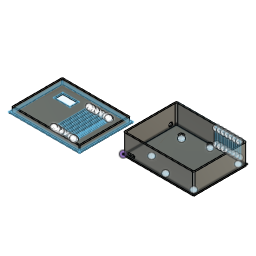
Enclosure temperature control box v10 (Autodesk Fusion 360 design; units mm, degrees)
Autodesk Fusion 360 part; units mm, degrees
sketch "Sketch1" plane through (0, 0, 0) normal (0, 0, 1) x (1, 0, 0)
  line L0 (0, 0) -> (110, 0)
  line L1 (110, 0) -> (110, 83)
  line L2 (110, 83) -> (0, 83)
  line L3 (0, 83) -> (0, 0)
  circle A0 centre (24.6, 66.3) radius 1.8
  circle A1 centre (24.6, 19.6) radius 1.8
  circle A2 centre (59.2, 6.8) radius 1.5
  circle A3 centre (103.2, 6.8) radius 1.5
  circle A4 centre (103.2, 76.2) radius 1.5
  circle A5 centre (59.2, 76.2) radius 1.5
  line L4 (2, 81) -> (108, 81)
  line L5 (108, 81) -> (108, 2)
  line L6 (108, 2) -> (2, 2)
  line L7 (2, 2) -> (2, 81)
  circle A6 centre (24.6, 66.3) radius 3.8
  circle A7 centre (24.6, 19.6) radius 3.8
  circle A8 centre (59.2, 76.2) radius 3.5
  circle A9 centre (103.2, 76.2) radius 3.5
  circle A10 centre (59.2, 6.8) radius 3.5
  circle A11 centre (103.2, 6.8) radius 3.5
  dimension "d1" = 110
  dimension "d2" = 83
  dimension "d10" = 3.6
  dimension "d13" = 3.6
  dimension "d16" = 3
  dimension "d19" = 3
  dimension "d22" = 3
  dimension "d25" = 3
  dimension "d28" = 106
  dimension "d29" = 79
  dimension "d30" = 2
  dimension "d31" = 2
  dimension "d40" = 7.6
  dimension "d41" = 7.6
  dimension "d42" = 7
  dimension "d43" = 7
  dimension "d44" = 7
  dimension "d45" = 7
  constraint horizontal L0
  constraint vertical L1
  constraint horizontal L2
  constraint vertical L3
  constraint coincident L0.start L3.end
  constraint horizontal L4
  constraint vertical L5
  constraint horizontal L6
  constraint vertical L7
  constraint concentric A0 A6
  constraint concentric A1 A7
  constraint concentric A5 A8
  constraint concentric A4 A9
  constraint concentric A2 A10
  constraint concentric A3 A11
  measures "d1" distance of L0.start L0.end
  measures "d2" distance of L0.start L2.end
  measures "d10" diameter of A0
  measures "d13" diameter of A1
  measures "d16" diameter of A2
  measures "d19" diameter of A3
  measures "d22" diameter of A4
  measures "d25" diameter of A5
  measures "d28" distance of L4.start L4.end
  measures "d29" distance of L4.start L6.end
  measures "d30" distance of L2 L4
  measures "d31" distance of L1 L5
  measures "d40" diameter of A6
  measures "d41" diameter of A7
  measures "d42" diameter of A8
  measures "d43" diameter of A9
  measures "d44" diameter of A10
  measures "d45" diameter of A11
extrude "Extrude4" add sketch "Sketch1" against normal blind 3 contours L0 L1 L2 L3 | A0 | A1 | A2 | A3 | A4 | A5 | L4 L5 L6 L7 | A6 | A7 | A8 | A9 | A10 | A11 makes body 1
extrude "Extrude5" add sketch "Sketch1" along normal blind 5 contours A6 | A7 | A8 | A9 | A10 | A11 bodies 1
extrude "Extrude6" add sketch "Sketch1" along normal blind 30 contours L0 L1 L2 L3 bodies 1
fillet "Fillet2" radius 2 4 edges at (110, 0, 13.5) (110, 83, 13.5) (0, 83, 13.5) (0, 0, 13.5) on bodies 1
fillet "Fillet3" radius 2 4 edges at (2, 2, 15) (108, 2, 15) (108, 81, 15) (2, 81, 15) on bodies 1
fillet "Fillet4" radius 1 8 edges at (109.4142, 82.4142, -3) (110, 41.5, -3) (109.4142, 0.5858, -3) (55, 0, -3) (0.5858, 0.5858, -3) (0, 41.5, -3) (0.5858, 82.4142, -3) (55, 83, -3) on bodies 1
sketch "Sketch2" plane through (0, 83, 0) normal (0, 1, 0) x (-1, 0, 0)
  line L0 (-108, -2) -> (-2, -2)
  line L1 (-2, -2) -> (-2, 30)
  line L2 (-2, 30) -> (-108, 30)
  line L3 (-108, 30) -> (-108, -2)
  line L4 (-97.0499, 25) -> (-97.0499, 3)
  line L5 (-100.0499, 3) -> (-100.0499, 25)
  arc A0 (-97.0499, 25) -> (-100.0499, 25) centre (-98.5499, 25) ccw
  arc A1 (-100.0499, 3) -> (-97.0499, 3) centre (-98.5499, 3) ccw
  line L6 (-94.0499, 3) -> (-94.0499, 25)
  line L7 (-91.0499, 25) -> (-91.0499, 3)
  arc A2 (-91.0499, 25) -> (-94.0499, 25) centre (-92.5499, 25) ccw
  arc A3 (-94.0499, 3) -> (-91.0499, 3) centre (-92.5499, 3) ccw
  line L8 (-88.0499, 3) -> (-88.0499, 25)
  line L9 (-85.0499, 25) -> (-85.0499, 3)
  arc A4 (-85.0499, 25) -> (-88.0499, 25) centre (-86.5499, 25) ccw
  arc A5 (-88.0499, 3) -> (-85.0499, 3) centre (-86.5499, 3) ccw
  line L10 (-82.0499, 3) -> (-82.0499, 25)
  line L11 (-79.0499, 25) -> (-79.0499, 3)
  arc A6 (-79.0499, 25) -> (-82.0499, 25) centre (-80.5499, 25) ccw
  arc A7 (-82.0499, 3) -> (-79.0499, 3) centre (-80.5499, 3) ccw
  line L12 (-76.0499, 3) -> (-76.0499, 25)
  line L13 (-73.0499, 25) -> (-73.0499, 3)
  arc A8 (-73.0499, 25) -> (-76.0499, 25) centre (-74.5499, 25) ccw
  arc A9 (-76.0499, 3) -> (-73.0499, 3) centre (-74.5499, 3) ccw
  line L14 (-70.0499, 3) -> (-70.0499, 25)
  line L15 (-67.0499, 25) -> (-67.0499, 3)
  arc A10 (-67.0499, 25) -> (-70.0499, 25) centre (-68.5499, 25) ccw
  arc A11 (-70.0499, 3) -> (-67.0499, 3) centre (-68.5499, 3) ccw
  line L16 (-64.0499, 3) -> (-64.0499, 25)
  line L17 (-61.0499, 25) -> (-61.0499, 3)
  arc A12 (-61.0499, 25) -> (-64.0499, 25) centre (-62.5499, 25) ccw
  arc A13 (-64.0499, 3) -> (-61.0499, 3) centre (-62.5499, 3) ccw
  dimension "d60" = 1.5
  dimension "d61" = 1.5
  dimension "d62" = 1.5
  dimension "d63" = 1.5
  dimension "d64" = 1.5
  dimension "d65" = 1.5
  dimension "d66" = 1.5
  dimension "d67" = 1.5
  dimension "d68" = 1.5
  dimension "d69" = 1.5
  dimension "d70" = 1.5
  dimension "d71" = 1.5
  dimension "d72" = 1.5
  dimension "d73" = 1.5
  dimension "d74" = 5
  dimension "d75" = 5
  dimension "d76" = 5
  dimension "d77" = 5
  dimension "d78" = 5
  dimension "d79" = 5
  dimension "d80" = 5
  dimension "d81" = 3
  dimension "d82" = 3
  dimension "d83" = 3
  dimension "d84" = 22
  dimension "d85" = 3
  dimension "d86" = 3
  dimension "d87" = 3
  constraint vertical L4
  constraint vertical L5
  constraint tangent L5 A0
  constraint tangent L4 A0
  constraint vertical L7
  constraint vertical L6
  constraint tangent L6 A2
  constraint tangent L7 A2
  constraint vertical L9
  constraint vertical L8
  constraint tangent L8 A4
  constraint tangent L9 A4
  constraint vertical L11
  constraint vertical L10
  constraint tangent L10 A6
  constraint tangent L11 A6
  constraint vertical L13
  constraint vertical L12
  constraint tangent L12 A8
  constraint tangent L13 A8
  constraint vertical L15
  constraint vertical L14
  constraint tangent L14 A10
  constraint tangent L15 A10
  constraint vertical L17
  constraint vertical L16
  constraint tangent L16 A12
  constraint tangent L17 A12
  measures "d60" radius of A0
  measures "d61" radius of A1
  measures "d62" radius of A2
  measures "d63" radius of A3
  measures "d64" radius of A4
  measures "d65" radius of A5
  measures "d66" radius of A6
  measures "d67" radius of A7
  measures "d68" radius of A8
  measures "d69" radius of A9
  measures "d70" radius of A10
  measures "d71" radius of A11
  measures "d72" radius of A12
  measures "d73" radius of A13
  measures "d74" distance of L2 A0.centre
  measures "d75" distance of L2 A2.centre
  measures "d76" distance of L2 A4.centre
  measures "d77" distance of L2 A6.centre
  measures "d78" distance of L2 A8.centre
  measures "d79" distance of L2 A10.centre
  measures "d80" distance of L2 A12.centre
  measures "d81" distance of L4 L6
  measures "d82" distance of L7 L8
  measures "d83" distance of L9 L10
  measures "d84" distance of L12.end L12.start
  measures "d85" distance of L11 L12
  measures "d86" distance of L13 L14
  measures "d87" distance of L15 L16
extrude "Extrude8" cut sketch "Sketch2" along normal mid plane 5.5 contours L4 L5 A0 A1 | L6 L7 A2 A3 | L8 L9 A4 A5 | L10 L11 A6 A7 | L12 L13 A8 A9 | L14 L15 A10 A11 | L16 L17 A12 A13 bodies 1
sketch "Sketch3" plane through (0, 0, 0) normal (0, 0, 1) x (1, 0, 0)
  line L0 (-146.1549, 50.841) -> (-36.1549, 50.841)
  line L1 (-36.1549, 50.841) -> (-36.1549, -32.159)
  line L2 (-36.1549, -32.159) -> (-146.1549, -32.159)
  line L3 (-146.1549, -32.159) -> (-146.1549, 50.841)
  line L4 (-144.1549, 48.841) -> (-38.1549, 48.841)
  line L5 (-38.1549, 48.841) -> (-38.1549, -30.159)
  line L6 (-38.1549, -30.159) -> (-144.1549, -30.159)
  line L7 (-144.1549, -30.159) -> (-144.1549, 48.841)
  line L8 (-142.1549, -28.159) -> (-40.1549, -28.159)
  line L9 (-40.1549, -28.159) -> (-40.1549, 46.841)
  line L10 (-40.1549, 46.841) -> (-142.1549, 46.841)
  line L11 (-142.1549, 46.841) -> (-142.1549, -28.159)
  line L12 (-60, -18.159) -> (-60, 36.841)
  arc A0 (-60, -18.159) -> (-56, -18.159) centre (-58, -18.159) ccw
  line L13 (-56, 36.841) -> (-56, -18.159)
  line L14 (-60, -18.159) -> (-60, 36.841)
  arc A1 (-56, 36.841) -> (-60, 36.841) centre (-58, 36.841) ccw
  arc A2 (-60, -18.159) -> (-56, -18.159) centre (-58, -18.159) ccw
  line L15 (-56, 36.841) -> (-56, -18.159)
  arc A3 (-56, 36.841) -> (-60, 36.841) centre (-58, 36.841) ccw
  arc A4 (-72.0861, -17.9826) -> (-68.0861, -17.9826) centre (-70.0861, -17.9826) ccw
  line L16 (-68.0861, 37.0174) -> (-68.0861, -17.9826)
  line L17 (-72.0861, -17.9826) -> (-72.0861, 37.0174)
  arc A5 (-68.0861, 37.0174) -> (-72.0861, 37.0174) centre (-70.0861, 37.0174) ccw
  arc A6 (-65.9979, -17.8944) -> (-61.9979, -17.8944) centre (-63.9979, -17.8944) ccw
  line L18 (-61.9979, 37.1056) -> (-61.9979, -17.8944)
  line L19 (-65.9979, -17.8944) -> (-65.9979, 37.1056)
  arc A7 (-61.9979, 37.1056) -> (-65.9979, 37.1056) centre (-63.9979, 37.1056) ccw
  arc A8 (-78.0818, -17.9826) -> (-74.0818, -17.9826) centre (-76.0818, -17.9826) ccw
  line L20 (-74.0818, 37.0174) -> (-74.0818, -17.9826)
  line L21 (-78.0818, -17.9826) -> (-78.0818, 37.0174)
  arc A9 (-74.0818, 37.0174) -> (-78.0818, 37.0174) centre (-76.0818, 37.0174) ccw
  line L22 (-60, -18.159) -> (-60, 36.841)
  line L23 (-80.3443, 36.9292) -> (-80.3443, -18.0708)
  line L24 (-84.3443, -18.0708) -> (-84.3443, 36.9292)
  arc A10 (-84.3443, -18.0708) -> (-80.3443, -18.0708) centre (-82.3443, -18.0708) ccw
  arc A11 (-80.3443, 36.9292) -> (-84.3443, 36.9292) centre (-82.3443, 36.9292) ccw
  line L25 (-86.5186, 37.0174) -> (-86.5186, -17.9826)
  line L26 (-90.5186, -17.9826) -> (-90.5186, 37.0174)
  arc A12 (-90.5186, -17.9826) -> (-86.5186, -17.9826) centre (-88.5186, -17.9826) ccw
  arc A13 (-86.5186, 37.0174) -> (-90.5186, 37.0174) centre (-88.5186, 37.0174) ccw
  line L27 (-129.9732, 35.4296) -> (-105.2732, 35.4296)
  line L28 (-105.2732, 35.4296) -> (-105.2732, 21.9296)
  line L29 (-105.2732, 21.9296) -> (-129.9732, 21.9296)
  line L30 (-129.9732, 21.9296) -> (-129.9732, 35.4296)
  dimension "d92" = 110
  dimension "d93" = 83
  dimension "d94" = 106
  dimension "d95" = 79
  dimension "d96" = 2
  dimension "d97" = 2
  dimension "d98" = 102
  dimension "d99" = 75
  dimension "d100" = 2
  dimension "d101" = 2
  dimension "d106" = 2
  dimension "d107" = 2
  dimension "d108" = 2
  dimension "d109" = 2
  dimension "d110" = 2
  dimension "d111" = 2
  dimension "d112" = 2
  dimension "d121" = 24.7
  dimension "d122" = 13.5
  constraint horizontal L0
  constraint vertical L1
  constraint horizontal L2
  constraint vertical L3
  constraint horizontal L4
  constraint vertical L5
  constraint horizontal L6
  constraint vertical L7
  constraint horizontal L8
  constraint vertical L9
  constraint horizontal L10
  constraint vertical L11
  constraint vertical L12
  constraint vertical L13
  constraint vertical L14
  constraint tangent L14 A1
  constraint tangent L13 A1
  constraint tangent A0 L14
  constraint tangent A0 L13
  constraint vertical L15
  constraint tangent L15 A3
  constraint tangent A2 L15
  constraint vertical L16
  constraint vertical L17
  constraint tangent L17 A5
  constraint tangent L16 A5
  constraint tangent A4 L17
  constraint tangent A4 L16
  constraint vertical L18
  constraint vertical L19
  constraint tangent L19 A7
  constraint tangent L18 A7
  constraint tangent A6 L19
  constraint tangent A6 L18
  constraint vertical L20
  constraint vertical L21
  constraint tangent L21 A9
  constraint tangent L20 A9
  constraint tangent A8 L21
  constraint tangent A8 L20
  constraint vertical L22
  constraint vertical L24
  constraint vertical L23
  constraint vertical L26
  constraint vertical L25
  constraint horizontal L27
  constraint vertical L28
  constraint horizontal L29
  constraint vertical L30
  measures "d92" distance of L0.start L0.end
  measures "d93" distance of L0.start L2.end
  measures "d94" distance of L4.start L4.end
  measures "d95" distance of L4.start L6.end
  measures "d96" distance of L0 L4
  measures "d97" distance of L3 L7
  measures "d98" distance of L8.start L8.end
  measures "d99" distance of L8.start L10.end
  measures "d100" distance of L4 L10
  measures "d101" distance of L7 L11
  measures "d106" radius of A1
  measures "d107" radius of A3
  measures "d108" radius of A5
  measures "d109" radius of A7
  measures "d110" radius of A9
  measures "d111" radius of A11
  measures "d112" radius of A13
  measures "d121" distance of L27.start L27.end
  measures "d122" distance of L27.start L29.end
extrude "Extrude9" add sketch "Sketch3" against normal blind 2 separate body contours L0 L1 L2 L3 | L4 L5 L6 L7 | L8 L9 L10 L11 | L27 L28 L29 L30 makes body 2
extrude "Extrude10" add sketch "Sketch3" along normal blind 7 contours L4 L5 L6 L7 bodies 2
fillet "Fillet5" radius 1 4 edges at (-91.1549, 50.841, -2) (-146.1549, 9.341, -2) (-91.1549, -32.159, -2) (-36.1549, 9.341, -2) on bodies 2
fillet "Fillet6" radius 1 4 edges at (-38.1549, -30.159, 3.5) (-144.1549, -30.159, 3.5) (-144.1549, 48.841, 3.5) (-38.1549, 48.841, 3.5) on bodies 2
extrude "Extrude11" cut sketch "Sketch3" along normal mid plane 6 contours L27 L28 L29 L30 bodies 2
sketch "Sketch4" plane through (0, 0, 0) normal (0, -1, 0) x (1, 0, 0)
  line L0 (2, -2) -> (108, -2)
  line L1 (108, -2) -> (108, 30)
  line L2 (108, 30) -> (2, 30)
  line L3 (2, 30) -> (2, -2)
  line L4 (9.4443, 6.4285) -> (16.0589, 6.4285)
  line L5 (16.0589, 2.4285) -> (9.4443, 2.4285)
  arc A0 (9.4443, 6.4285) -> (9.4443, 2.4285) centre (9.4443, 4.4285) ccw
  arc A1 (16.0589, 2.4285) -> (16.0589, 6.4285) centre (16.0589, 4.4285) ccw
  dimension "d127" = 2
  constraint horizontal L4
  constraint horizontal L5
  constraint tangent L4 A0
  constraint tangent L5 A0
  constraint tangent L4 A1
  constraint tangent L5 A1
  measures "d127" radius of A0
extrude "Extrude12" cut sketch "Sketch4" along normal mid plane 6 contours L4 L5 A0 A1 bodies 1
sketch "Sketch5" plane through (0, 0, 0) normal (-1, 0, 0) x (0, -1, 0)
  line L0 (-81, -2) -> (-2, -2)
  line L1 (-2, -2) -> (-2, 30)
  line L2 (-2, 30) -> (-81, 30)
  line L3 (-81, 30) -> (-81, -2)
  circle A0 centre (-72.1769, 4.9272) radius 3
  dimension "d130" = 6
  measures "d130" diameter of A0
extrude "Extrude13" cut sketch "Sketch5" along normal mid plane 6 contours A0 bodies 1
fillet "Fillet7" radius 1 4 edges at (-40.1549, 46.841, 3.5) (-40.1549, -28.159, 3.5) (-142.1549, 46.841, 3.5) (-142.1549, -28.159, 3.5) on bodies 2
extrude "Extrude7" [suppressed]
extrude "Extrude1" [suppressed]
extrude "Extrude2" [suppressed]
extrude "Extrude3" [suppressed]
fillet "Fillet1" [suppressed]
